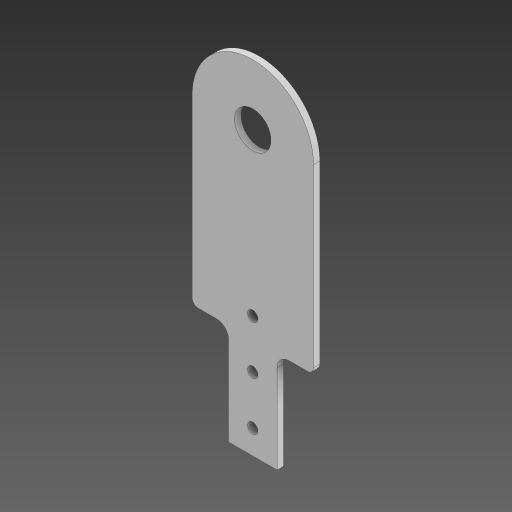
# Autodesk Inventor part: Wrist plate
Saved by Autodesk Inventor 2024 (Build 280153000, 153)
## iProperties
Created: 2023-11-02
Part Number: Wrist plate
Material: Generic
Document SubType Name: Modeling
Designer: ellen
Density: 1 g/cm^3
Appearance: Default
Author: ellen
Autodesk Inventor part; units mm, degrees
ref_plane "YZ Plane" through (0, 0, 0) normal (1, 0, 0) x (0, 1, 0)
ref_plane "XZ Plane" through (0, 0, 0) normal (0, 1, 0) x (-1, 0, 0)
ref_plane "XY Plane" through (0, 0, 0) normal (0, 0, 1) x (1, 0, 0)
sketch "Sketch1" plane through (0, 0, 0) normal (0, 0, 1) x (1, 0, 0)
  line L0 (0, 0) -> (63.5, 0)
  line L1 (63.5, 0) -> (63.5, 127)
  line L2 (63.5, 127) -> (0, 127)
  line L3 (0, 127) -> (0, 0)
  circle A0 centre (31.75, 95.25) radius 9.5
  circle A1 centre (31.75, 10.795) radius 2.6543
  circle A2 centre (31.75, -14.605) radius 2.6543
  line L4 (31.75, 115.6989) -> (31.75, 0)
  circle A3 centre (31.75, -40.005) radius 2.6543
  line L5 (44.45, 39.5543) -> (44.45, -52.705)
  line L6 (44.45, -52.705) -> (19.05, -52.705)
  line L7 (19.05, -52.705) -> (19.05, 39.5543)
  line L8 (44.45, 39.5543) -> (19.05, 39.5543)
  line L9 (0, 30.254) -> (63.5, 30.254)
  point P0 (44.45, 0)
  point P1 (19.05, 0)
  point P2 (31.75, -52.705)
  dimension "d0" = 63.5
  dimension "d1" = 127
  dimension "d2" = 19
  dimension "d3" = 5.3086
  dimension "d4" = 5.3086
  dimension "d5" = 31.75
  dimension "d6" = 116.205
  dimension "d14" = 25.4
  dimension "d15" = 25.4
  dimension "d17" = 25.4
  dimension "d20" = 39.5543
  dimension "d21" = 12.7
  constraints: 20 end point, 4 centre point, 4 perpendicular, 2 horizontal, 2 midpoint, 2 parallel, 2 point on line, 1 equal radius, 1 other
  measures "d0" distance of L2.end L1.end
  measures "d1" distance of L1.end L0.end
  measures "d2" diameter of A0
  measures "d3" diameter of A1
  measures "d4" diameter of A2
  measures "d5" distance from line of A0.centre L2
  measures "d6" distance from line of L2 A1.centre
  measures "d14" distance of A2.centre A1.centre
  measures "d15" distance of A3.centre A2.centre
  measures "d17" distance of L5.end L6.end
  measures "d20" distance between parallel lines of L0 L8
  measures "d21" distance of point (31.75, -52.705) A3.centre
extrude "Extrusion1" add sketch "Sketch1" along normal blind 3.302 contours L3 L9 L7 L0 | L7 L9 L4 A1 L0 | L0 L5 L6 L7 | L3 L2 L1 L9 L5 L8 L7 | L4 A1 L9 L5 L0 | L7 L8 L4 L9 | L5 L9 L1 L0 | L4 L8 L5 L9
fillet "Fillet1" radius 31.75 1 edges at (63.5, 127, 1.651)
fillet "Fillet2" radius 31.75 1 edges at (0, 127, 1.651)
fillet "Fillet3" radius 3.175 1 edges at (63.5, 0, 1.651)
fillet "Fillet4" radius 3.175 1 edges at (0, 0, 1.651)
fillet "Fillet5" radius 6.35 2 edges at (19.05, 0, 1.651) (44.45, 0, 1.651)
body "Solid1"
